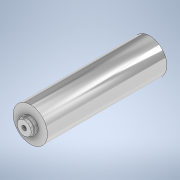
# Autodesk Inventor part: 38120s-10Ah
Saved by Autodesk Inventor 2022 (Build 260153000, 153)
## iProperties
Company: El Camino College
Created: 2022-12-17
Part Number: 38120s-10Ah
Material: Nickel-Copper Alloy 400
Document SubType Name: Modeling
Designer: Edgar Tejada
Density: 8.83 g/cm^3
Appearance: Chrome - Polished
Project: Parametric-Modeling
Author: Edgar Tejada
Title: Battery 38120s-10Ah
Autodesk Inventor part; units mm, degrees
ref_plane "YZ Plane" through (0, 0, 0) normal (1, 0, 0) x (0, 1, 0)
ref_plane "XZ Plane" through (0, 0, 0) normal (0, 1, 0) x (-1, 0, 0)
ref_plane "XY Plane" through (0, 0, 0) normal (0, 0, 1) x (1, 0, 0)
sketch "Sketch1" plane through (0, 0, 0) normal (0, 0, 1) x (1, 0, 0)
  circle A0 centre (0, 0) radius 19
  dimension "d0" = 38
  constraints: 1 centre point, 1 coincident
  measures "d0" diameter of A0
extrude "Base_Shell" add sketch "Sketch1" along normal mid plane 132
sketch "Sketch2" plane through (0, 0, 66) normal (0, 0, 1) x (1, 0, 0)
  circle A0 centre (0, 0) radius 8.75
  dimension "d3" = 17.5
  constraints: 1 centre point, 1 coincident
  measures "d3" diameter of A0
extrude "Terminal_Shell" add sketch "Sketch2" along normal blind 3.8
sketch "Sketch3" plane through (0, 0, 69.8) normal (0, 0, 1) x (1, 0, 0)
  circle A0 centre (0, 0) radius 7.75
  dimension "d6" = 15.5
  constraints: 1 centre point, 1 coincident
  measures "d6" diameter of A0
extrude "Terminal" add sketch "Sketch3" along normal blind 3
sketch "Sketch4" plane through (0, 0, 72.8) normal (0, 0, 1) x (1, 0, 0)
  circle A0 centre (0, 0) radius 2.5
  dimension "d9" = 5
  constraints: 1 centre point, 1 coincident
  measures "d9" diameter of A0
extrude "M5_Terminal_Screw_hole" cut sketch "Sketch4" against normal blind 5
mirror "Mirror1" about plane through (0, 0, 0) normal (0, 0, 1) of "Terminal_Shell", "Terminal", "M5_Terminal_Screw_hole"
equation "\"d1\" = 3.47368 * d0"
equation "\"d3\" = 0.460526 * d0"
equation "\"d4\" = 0.1 * d0"
equation "\"d6\" = 0.407895 * d0"
equation "\"d7\" = 0.0789474 * d0"
equation "\"d9\" = 0.131579 * d0"
equation "\"d10\" = d9"
body "Solid1"
